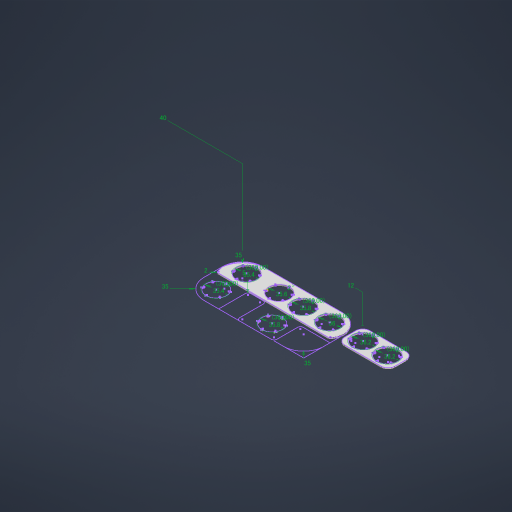
# Autodesk Inventor part: template
Saved by Autodesk Inventor 2024.3 (Build 283343000, 343)
## iProperties
Created: 2025-03-03
Part Number: template
Material: 一般
Document SubType Name: Sheet Metal
Designer: ktamu
Density: 1 g/cm^3
Sheet Metal Rule: Default_mm
Appearance: 既定
Author: ktamu
Autodesk Inventor part; units mm, degrees
ref_plane "YZ Plane" through (0, 0, 0) normal (1, 0, 0) x (0, 1, 0)
ref_plane "XZ Plane" through (0, 0, 0) normal (0, 1, 0) x (-1, 0, 0)
ref_plane "XY Plane" through (0, 0, 0) normal (0, 0, 1) x (1, 0, 0)
sketch "BASEsc" plane through (0, 0, 0) normal (0, 1, 0) x (-1, 0, 0)
  arc A0 (-30.7364, -0.0681) -> (-28.0904, 4.5242) centre (-30.3216, 2.7513) ccw
  arc A1 (-16.8277, 11.04) -> (-11.5277, 11.0446) centre (-14.1786, 12.0904) ccw
  arc A2 (-11.4967, -24.1586) -> (-16.7967, -24.1633) centre (-14.1458, -25.2091) ccw
  arc A3 (-0.2535, 4.5487) -> (2.4005, -0.0389) centre (1.9807, 2.7798) ccw
  arc A4 (-28.0709, -17.6674) -> (-30.7249, -13.0798) centre (-30.3051, -15.8984) ccw
  circle A5 centre (-14.1622, -6.5593) radius 17.8
  arc A6 (2.412, -13.0506) -> (-0.234, -17.6429) centre (1.9972, -15.87) ccw
  circle A7 centre (-55.7283, -6.3362) radius 17.9
  arc A8 (-58.3938, 11.2631) -> (-53.0938, 11.2678) centre (-55.7447, 12.3136) ccw
  arc A9 (-41.8196, 4.7719) -> (-39.1656, 0.1843) centre (-39.5854, 3.0029) ccw
  arc A10 (-72.3025, 0.1551) -> (-69.6565, 4.7474) centre (-71.8877, 2.9745) ccw
  arc A11 (-69.637, -17.4442) -> (-72.291, -12.8566) centre (-71.8712, -15.6753) ccw
  arc A12 (-53.0767, -24.0387) -> (-58.3776, -24.039) centre (-55.7271, -25.0859) ccw
  arc A13 (-39.1541, -12.8274) -> (-41.8001, -17.4197) centre (-39.569, -15.6468) ccw
  circle A14 centre (-101.6822, -6.2265) radius 18
  arc A15 (-99.0445, -24.0322) -> (-104.3463, -24.0282) centre (-101.6962, -25.0761) ccw
  arc A16 (-39.0717, -12.8911) -> (-41.7218, -17.4819) centre (-39.49, -15.71) ccw
  arc A17 (-41.7233, 4.8114) -> (-39.0725, 0.2209) centre (-39.4912, 3.0397) ccw
  arc A18 (-58.3799, 11.3664) -> (-53.079, 11.3667) centre (-55.7295, 12.4135) ccw
  arc A19 (-72.3849, 0.2188) -> (-69.7348, 4.8096) centre (-71.9666, 3.0377) ccw
  arc A20 (-69.7334, -17.4837) -> (-72.3841, -12.8932) centre (-71.9654, -15.7121) ccw
  circle A21 centre (43.1966, -7.3809) radius 17.7
  arc A22 (45.8761, -24.8769) -> (40.5769, -24.886) centre (43.2283, -25.9306) ccw
  circle A23 centre (45.2732, 42.9601) radius 17.7
  arc A24 (47.7889, 25.4398) -> (42.6535, 25.455) centre (45.2175, 24.2112) ccw
  arc A25 (-51.2492, 27.6525) -> (-56.3871, 27.6758) centre (-53.8237, 26.4307) ccw
  circle A26 centre (-53.7378, 45.3786) radius 17.9
  arc A27 (-84.9432, -12.845) -> (-87.5975, -17.4345) centre (-85.365, -15.6634) ccw
  arc A28 (-87.5809, 4.9607) -> (-84.9334, 0.3672) centre (-85.351, 3.1862) ccw
  arc A29 (-104.3199, 11.5792) -> (-99.0181, 11.5753) centre (-101.6682, 12.6231) ccw
  arc A30 (-118.4212, 0.3921) -> (-115.7669, 4.9816) centre (-117.9994, 3.2104) ccw
  arc A31 (-115.7835, -17.4136) -> (-118.431, -12.8202) centre (-118.0134, -15.6392) ccw
  arc A32 (-37.1422, 38.6707) -> (-39.7313, 34.2328) centre (-37.3714, 35.8302) ccw
  arc A33 (-39.6308, 56.3969) -> (-37.082, 51.9357) centre (-37.2854, 54.7782) ccw
  arc A34 (-56.2264, 63.1048) -> (-51.0885, 63.0815) centre (-53.6518, 64.3265) ccw
  arc A35 (-70.3334, 52.0865) -> (-67.7443, 56.5244) centre (-70.1042, 54.927) ccw
  arc A36 (-67.8448, 34.3603) -> (-70.3936, 38.8215) centre (-70.1901, 35.9791) ccw
  arc A37 (61.7041, 36.3785) -> (59.1232, 31.9388) centre (61.4824, 33.5374) ccw
  arc A38 (59.1885, 53.8989) -> (61.7429, 49.4439) centre (61.5381, 52.2863) ccw
  arc A39 (42.7576, 60.4804) -> (47.8929, 60.4652) centre (45.3289, 61.7089) ccw
  arc A40 (28.8424, 49.5417) -> (31.4233, 53.9813) centre (29.0641, 52.3828) ccw
  arc A41 (31.358, 32.0213) -> (28.8036, 36.4763) centre (29.0084, 33.6339) ccw
  arc A42 (59.6883, -13.8084) -> (57.0466, -18.4022) centre (59.2769, -16.6283) ccw
  arc A43 (57.0088, 3.6876) -> (59.6663, -0.8971) centre (59.2452, 1.9214) ccw
  arc A44 (40.5171, 10.1151) -> (45.8163, 10.1242) centre (43.1649, 11.1688) ccw
  arc A45 (26.7049, -0.9534) -> (29.3466, 3.6404) centre (27.1162, 1.8665) ccw
  arc A46 (29.3843, -18.4494) -> (26.7269, -13.8647) centre (27.1479, -16.6832) ccw
  line L0 (39.5339, -31.8115) -> (-97.6905, -31.8115)
  line L1 (-132.6905, 3.1885) -> (-132.6905, 34.7246)
  line L2 (-76.3868, 69.7246) -> (-21.7967, 69.7246)
  line L3 (74.5339, 34.7246) -> (74.5339, 3.1885)
  arc A47 (34.5339, -31.8115) -> (74.5339, 8.1885) centre (34.5339, 8.1885) ccw
  arc A48 (74.5339, 34.7246) -> (39.5339, 69.7246) centre (39.5339, 34.7246) ccw
  arc A49 (39.5339, -31.8115) -> (74.5339, 3.1885) centre (39.5339, 3.1885) ccw
  arc A50 (-132.6905, 3.1885) -> (-97.6905, -31.8115) centre (-97.6905, 3.1885) ccw
  arc A51 (-97.6905, 69.7246) -> (-132.6905, 34.7246) centre (-97.6905, 34.7246) ccw
  line L4 (-86.3868, 24.2112) -> (-132.6905, 24.2112)
  line L5 (-132.6905, 24.2112) -> (-132.6905, 69.7246)
  line L6 (-132.6905, 69.7246) -> (-81.3868, 69.7246)
  line L7 (-81.3868, 64.7246) -> (-81.3868, 29.2112)
  line L8 (14.5191, 69.7246) -> (-16.7967, 69.7246)
  line L9 (-16.7967, 64.7246) -> (-16.7967, 23.9565)
  line L10 (-11.7967, 18.9565) -> (9.5191, 18.9565)
  line L11 (14.5191, 23.9565) -> (14.5191, 69.7246)
  arc A52 (9.5191, 18.9565) -> (14.5191, 23.9565) centre (9.5191, 23.9565) ccw
  arc A53 (-16.7967, 23.9565) -> (-11.7967, 18.9565) centre (-11.7967, 23.9565) ccw
  arc A54 (-86.3868, 24.2112) -> (-81.3868, 29.2112) centre (-86.3868, 29.2112) ccw
  arc A55 (-76.3868, 69.7246) -> (-81.3868, 64.7246) centre (-76.3868, 64.7246) ccw
  arc A56 (-16.7967, 64.7246) -> (-21.7967, 69.7246) centre (-21.7967, 64.7246) ccw
  line L12 (39.5339, 69.7246) -> (-21.7967, 69.7246)
  line L13 (74.5339, 3.1885) -> (71.4874, 14.7614)
  line L14 (69.5661, 16.2522) -> (-124.7088, 17.4921)
  line L15 (-126.5328, 16.3402) -> (-132.6905, 3.1885)
  arc A57 (71.4874, 14.7614) -> (69.5661, 16.2522) centre (69.5533, 14.2523) ccw
  arc A58 (-124.7088, 17.4921) -> (-126.5328, 16.3402) centre (-124.7215, 15.4921) ccw
  circle A59 centre (-159.085, -7.0568) radius 18.1
  arc A60 (-156.4662, -24.9663) -> (-161.7151, -24.9646) centre (-159.091, -25.965) ccw
  arc A61 (-142.2654, -13.7436) -> (-144.8914, -18.2885) centre (-142.7129, -16.5161) ccw
  arc A62 (-144.8843, 4.166) -> (-142.2612, -0.3806) centre (-142.7069, 2.3922) ccw
  arc A63 (-161.7038, 10.8528) -> (-156.4548, 10.8511) centre (-159.079, 11.8515) ccw
  arc A64 (-175.9045, -0.3699) -> (-173.2786, 4.175) centre (-175.457, 2.4026) ccw
  arc A65 (-173.2857, -18.2795) -> (-175.9087, -13.7329) centre (-175.463, -16.5057) ccw
  arc A66 (-186.9214, 4.5357) -> (-184.2983, -0.0109) centre (-184.744, 2.7619) ccw
  arc A67 (-203.7409, 11.2225) -> (-198.4919, 11.2208) centre (-201.1161, 12.2212) ccw
  arc A68 (-217.9416, -0.0003) -> (-215.3157, 4.5446) centre (-217.4942, 2.7723) ccw
  arc A69 (-215.3228, -17.9098) -> (-217.9458, -13.3632) centre (-217.5001, -16.136) ccw
  arc A70 (-198.5033, -24.5966) -> (-203.7522, -24.595) centre (-201.1281, -25.5954) ccw
  circle A71 centre (-201.1221, -6.6871) radius 18.1
  arc A72 (-184.3026, -13.3739) -> (-186.9285, -17.9188) centre (-184.75, -16.1464) ccw
  line L16 (-148.8172, -28.4145) -> (-211.9772, -28.4145)
  line L17 (-223.9772, -16.4145) -> (-223.9772, 2.858)
  line L18 (-211.9772, 14.858) -> (-148.8172, 14.858)
  line L19 (-136.8172, 2.858) -> (-136.8172, -16.4145)
  arc A73 (-148.8172, -28.4145) -> (-136.8172, -16.4145) centre (-148.8172, -16.4145) ccw
  arc A74 (-223.9772, -16.4145) -> (-211.9772, -28.4145) centre (-211.9772, -16.4145) ccw
  arc A75 (-211.9772, 14.858) -> (-223.9772, 2.858) centre (-211.9772, 2.858) ccw
  arc A76 (-136.8172, 2.858) -> (-148.8172, 14.858) centre (-148.8172, 2.858) ccw
  point P0 (0, 0)
  point P1 (-14.1467, -24.3593)
  point P2 (-27.8531, 1.3272)
  point P3 (-14.1777, 9.2407)
  point P4 (-14.1467, -22.3593)
  point P5 (-0.4868, 1.3541)
  point P6 (-27.8376, -14.4728)
  point P7 (-0.4712, -14.4459)
  point P8 (-41.5661, 0.2232)
  point P9 (-55.7127, -24.2361)
  point P10 (-55.7438, 9.4638)
  point P11 (-42.0529, 1.5773)
  point P12 (-69.4193, 1.5504)
  point P13 (-69.4038, -14.2496)
  point P14 (-55.7127, -22.2361)
  point P15 (-42.0374, -14.2227)
  point P16 (-87.52, 0.3329)
  point P17 (-101.6665, -24.2265)
  point P18 (-101.6977, 9.5735)
  point P19 (-88.0068, 1.6869)
  point P20 (-115.3732, 1.6601)
  point P21 (-115.3576, -14.1399)
  point P22 (-101.6665, -22.2265)
  point P23 (-87.9913, -14.1131)
  point P24 (-41.9507, -14.2726)
  point P25 (-41.9663, 1.6273)
  point P26 (-55.7439, 9.5638)
  point P27 (-69.5059, 1.6003)
  point P28 (-69.4903, -14.2997)
  point P29 (57.3588, -0.8216)
  point P30 (29.5211, -15.2943)
  point P31 (56.872, 0.5325)
  point P32 (43.212, -25.0809)
  point P33 (29.5056, 0.5057)
  point P34 (43.1811, 8.4191)
  point P35 (56.8875, -15.2675)
  point P36 (43.212, -23.0809)
  point P37 (59.4354, 49.5194)
  point P38 (31.5978, 35.0467)
  point P39 (58.9487, 50.8735)
  point P40 (45.2887, 25.2601)
  point P41 (31.5823, 50.8467)
  point P42 (45.2577, 58.7601)
  point P43 (58.9642, 35.0735)
  point P44 (45.2887, 27.0601)
  point P45 (-40.0468, 37.492)
  point P46 (-39.5756, 51.9379)
  point P47 (-40.0623, 53.292)
  point P48 (-53.7222, 29.2786)
  point P49 (-53.7222, 27.4786)
  point P50 (-53.7533, 61.1786)
  point P51 (-67.4287, 53.2652)
  point P52 (-67.4132, 37.4652)
  point P53 (-87.818, -14.2129)
  point P54 (-87.8336, 1.7871)
  point P55 (-101.6979, 9.7735)
  point P56 (-115.5464, 1.7599)
  point P57 (-115.5308, -14.2401)
  point P58 (-39.787, 37.3421)
  point P59 (-39.8026, 53.4421)
  point P60 (-53.7534, 61.4786)
  point P61 (-67.6886, 53.4151)
  point P62 (-67.673, 37.3151)
  point P63 (59.0507, 35.0234)
  point P64 (59.0353, 50.9234)
  point P65 (45.2578, 58.8601)
  point P66 (31.4957, 50.8967)
  point P67 (31.5111, 34.9967)
  point P68 (56.8009, -15.2175)
  point P69 (56.7855, 0.4824)
  point P70 (43.1812, 8.3191)
  point P71 (29.5923, 0.4557)
  point P72 (29.6077, -15.2442)
  point P73 (-97.6905, 69.7246)
  point P74 (-16.7967, 69.7246)
  point P75 (-67.8448, 34.3603)
  point P76 (-39.7313, 34.2328)
  point P77 (-37.1422, 38.6707)
  point P78 (-37.082, 51.9357)
  point P79 (-51.0885, 63.0815)
  point P80 (-67.7443, 56.5244)
  point P81 (-70.3334, 52.0865)
  point P82 (-118.431, -12.8202)
  point P83 (-115.7835, -17.4136)
  point P84 (-87.5975, -17.4345)
  point P85 (-84.9334, 0.3672)
  point P86 (-87.5809, 4.9607)
  point P87 (-104.3199, 11.5792)
  point P88 (-115.7669, 4.9816)
  point P89 (-118.4212, 0.3921)
  point P90 (-72.3841, -12.8932)
  point P91 (-39.0725, 0.2209)
  point P92 (-41.7233, 4.8114)
  point P93 (-53.079, 11.3667)
  point P94 (-58.3799, 11.3664)
  point P95 (-69.7348, 4.8096)
  point P96 (-72.3849, 0.2188)
  point P97 (-0.234, -17.6429)
  point P98 (2.412, -13.0506)
  point P99 (2.4005, -0.0389)
  point P100 (-0.2535, 4.5487)
  point P101 (-11.5277, 11.0446)
  point P102 (-16.8277, 11.04)
  point P103 (-28.0904, 4.5242)
  point P104 (-30.7364, -0.0681)
  point P105 (-28.0709, -17.6674)
  point P106 (29.3843, -18.4494)
  point P107 (59.6883, -13.8084)
  point P108 (59.6663, -0.8971)
  point P109 (57.0088, 3.6876)
  point P110 (40.5171, 10.1151)
  point P111 (29.3466, 3.6404)
  point P112 (26.7049, -0.9534)
  point P113 (47.8929, 60.4652)
  point P114 (31.4233, 53.9813)
  point P115 (28.8424, 49.5417)
  point P116 (74.3158, 4.017)
  point P117 (-144.9228, -0.4974)
  point P118 (-172.7604, -14.9702)
  point P119 (-145.4095, 0.8567)
  point P120 (-159.069, -25.1567)
  point P121 (-172.7759, 0.8298)
  point P122 (-159.1005, 8.7432)
  point P123 (-145.394, -14.9433)
  point P124 (-159.0676, -23.1567)
  point P125 (-145.1333, -15.0917)
  point P126 (-145.1507, 1.0083)
  point P127 (-159.1023, 9.0432)
  point P128 (-173.0367, 0.9782)
  point P129 (-173.0193, -15.1218)
  point P130 (-155.0933, 2.3582)
  point P131 (-186.9599, -0.1277)
  point P132 (-187.4466, 1.2264)
  point P133 (-214.7975, -14.6005)
  point P134 (-187.1878, 1.378)
  point P135 (-201.1394, 9.4129)
  point P136 (-215.0738, 1.3479)
  point P137 (-215.0564, -14.7521)
  point P138 (-187.4311, -14.5736)
  point P139 (-201.1376, 9.1129)
  point P140 (-201.1061, -24.7871)
  point P141 (-201.1047, -22.7871)
  point P142 (-214.813, 1.1995)
  point P143 (-187.1704, -14.722)
  point P144 (-197.1304, 2.7279)
  dimension "d0" = 35.6
  dimension "d1" = 2
  dimension "d2" = 35.8
  dimension "d3" = 2
  dimension "d4" = 36
  dimension "d5" = 2
  dimension "d8" = 360
  dimension "d10" = 35.4
  dimension "d11" = 2
  dimension "d12" = 35.4
  dimension "d13" = 1.8
  dimension "d14" = 35.8
  dimension "d15" = 1.8
  dimension "d18" = 360
  dimension "d22" = 360
  dimension "d26" = 360
  dimension "d30" = 360
  dimension "d32" = 40
  dimension "d33" = 35
  dimension "d34" = 35
  dimension "d35" = 35
  dimension "d36" = 5
  dimension "d46" = 2
  dimension "d51" = 36.2
  dimension "d52" = 2
  dimension "d53" = 360
  dimension "d56" = 36.2
  dimension "d57" = 2
  dimension "d58" = 360
  dimension "d59" = 12
  constraints: 215 point on circle, 77 centre point, 40 end point, 33 tangent, 9 equal radius, 8 parallel, 8 point on line, 5 horizontal, 4 perpendicular, 217 other
  measures "d0" diameter of A5
  measures "d1" distance of A5.start point (-14.147, -22.359)
  measures "d2" diameter of A7
  measures "d3" distance of A7.start point (-55.713, -22.236)
  measures "d4" diameter of A14
  measures "d5" distance of A14.start point (-101.667, -22.226)
  measures "d10" diameter of A21
  measures "d11" distance of A21.start point (43.212, -23.081)
  measures "d12" diameter of A23
  measures "d13" distance of A23.start point (45.289, 27.06)
  measures "d14" diameter of A26
  measures "d15" distance of A26.start point (-53.722, 29.279)
  measures "d32" radius of A47
  measures "d33" radius of A48
  measures "d34" radius of A49
  measures "d35" radius of A51
  measures "d36" radius of A52
  measures "d46" radius of A57
  measures "d51" diameter of A59
  measures "d52" distance of A59.start point (-159.068, -23.157)
  measures "d56" diameter of A71
  measures "d57" distance of A71.start point (-201.105, -22.787)
  measures "d59" radius of A73
extrude "押し出し1" add sketch "BASEsc" against normal blind 2.5 contours A5 A0 | A0 A5 A1 A3 A6 A2 A4 | A4 A5 | A5 A1 | A2 A5 | A5 A3 | A6 A5 | A7 A16 A12 A20 A19 A18 A17 | A17 A7 | A7 A16 | A18 A7 | A7 A12 | A19 A7 | A7 A20 | A14 A27 A15 A31 A30 A29 A28 | A28 A14 | A14 A27 | A29 A14 | A14 A15 | A30 A14 | A14 A31 | A21 A42 A22 A46 A45 A44 A43 | A43 A21 | A21 A42 | A44 A21 | A21 A22 | A45 A21 | A21 A46 | A23 A37 A24 A41 A40 A39 A38 | A38 A23 | A23 A37 | A39 A23 | A23 A24 | A40 A23 | A23 A41 | A26 A25 | A25 A26 A36 A35 A34 A33 A32 | A32 A26 | A26 A36 | A26 A35 | A33 A26 | A26 A34 | L0 A47 L13 A49 | L0 A50 L15 A58 L14 A57 L13 A47 | L13 A47 L3 | L13 A57 L14 A58 L15 L1 L4 A54 L7 A55 L2 A56 L9 A53 L10 A52 L11 L12 A48 L3 A47 | L11 A52 L10 A53 L9 A56 L12 L8 | A51 L5 L6
extrude "押し出し2" cut sketch "BASEsc" against normal through all contours A0 A5 A1 A3 A6 A2 A4 | A7 A16 A12 A20 A19 A18 A17 | A14 A27 A15 A31 A30 A29 A28 | A21 A42 A22 A46 A45 A44 A43 | A23 A37 A24 A41 A40 A39 A38 | A25 A26 A36 A35 A34 A33 A32
extrude "押し出し3" cut sketch "BASEsc" against normal blind 10 contours L11 A52 L10 A53 L9 A56 L12 L8 | A51 L5 L6
fillet "フィレット1" radius 25 1 edges at (132.6905, -1.25, 24.2112)
extrude "押し出し4" cut sketch "BASEsc" against normal blind 10 contours A5 A0 | A4 A5 | A5 A1 | A2 A5 | A5 A3 | A6 A5 | A17 A7 | A7 A16 | A18 A7 | A7 A12 | A19 A7 | A7 A20 | A28 A14 | A14 A27 | A29 A14 | A14 A15 | A30 A14 | A14 A31 | A43 A21 | A21 A42 | A44 A21 | A21 A22 | A45 A21 | A21 A46 | A38 A23 | A23 A37 | A39 A23 | A23 A24 | A40 A23 | A23 A41
extrude "押し出し5" cut sketch "BASEsc" against normal blind 10 contours L13 A57 L14 A58 L15 L1 L4 A54 L7 A55 L2 A56 L9 A53 L10 A52 L11 L12 A48 L3 A47
extrude "押し出し6" add sketch "BASEsc" against normal blind 2.5 contours L16 A74 L17 A75 L18 A76 L19 A73
equation "\"GapSize\" = Thickness"
equation "\"BendRadius\" = Thickness"
equation "\"MinimumRemnant\" = 2 * Thickness"
equation "\"BendReliefDepth\" = 0.5 * Thickness"
equation "\"BendReliefWidth\" = Thickness"
equation "\"CornerReliefSize\" = 4 * Thickness"
equation "\"JacobiRadiusSize\" = BendRadius"
equation "\"TransitionRadius\" = BendRadius"
equation "\"Thickness\" = 0.5"
